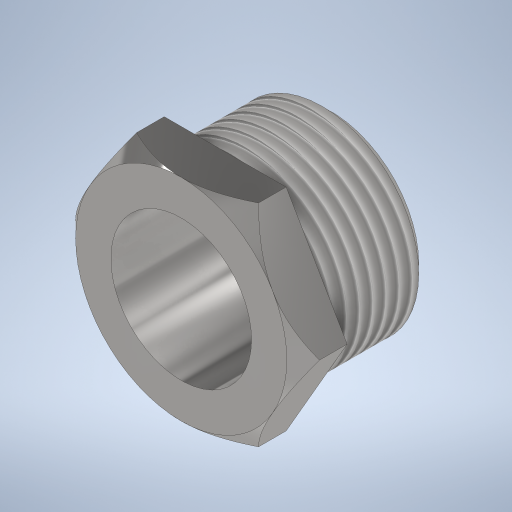
# Autodesk Inventor part: Hex.nut
Saved by Autodesk Inventor 2024 (Build 280153000, 153)
## iProperties
Created: 2024-03-04
Part Number: Hex.nut
Material: Generic
Document SubType Name: Sheet Metal
Designer: MSI-C
Density: 1 g/cm^3
Sheet Metal Rule: Default_mm
Appearance: Steel - Polished
Mass: 3.57819 g
Surface Area: 26.1963 cm^2
Volume: 3.57819 cm^3
Author: MSI-C
Autodesk Inventor part; units mm, degrees
ref_plane "YZ Plane" through (0, 0, 0) normal (1, 0, 0) x (0, 1, 0)
ref_plane "XZ Plane" through (0, 0, 0) normal (0, 1, 0) x (-1, 0, 0)
ref_plane "XY Plane" through (0, 0, 0) normal (0, 0, 1) x (1, 0, 0)
sketch "Sketch1" plane through (0, 0, 0) normal (0, 0, 1) x (1, 0, 0)
  line L0 (-6.9282, -12) -> (-13.8564, 0)
  line L1 (-13.8564, 0) -> (-6.9282, 12)
  line L2 (-6.9282, 12) -> (6.9282, 12)
  line L3 (6.9282, 12) -> (13.8564, 0)
  line L4 (13.8564, 0) -> (6.9282, -12)
  line L5 (6.9282, -12) -> (-6.9282, -12)
  circle A0 centre (0, 0) radius 12
  circle A1 centre (0, 0) radius 7
  dimension "d0" = 24
  dimension "d1" = 24
  dimension "d2" = 14
  constraints: 12 end point, 3 coincident, 2 centre point, 1 horizontal, 13 other
  measures "d0" distance between parallel lines of L5 L2
  measures "d1" diameter of A0
  measures "d2" diameter of A1
extrude "Extrusion1" add sketch "Sketch1" along normal blind 5 contours L0 A0 L5 | L0 L1 A0 | A0 | A0 L4 L5 | L1 L2 A0 | A0 L3 L4 | L2 L3 A0 | A1
sketch "Sketch2" plane through (0, 0, 5) normal (0, 0, 1) x (1, 0, 0)
  circle A0 centre (0, 0) radius 12
  dimension "d5" = 24
  constraints: 1 centre point, 1 coincident
  measures "d5" diameter of A0
extrude "Extrusion2" cut sketch "Sketch2" against normal blind 5 draft 45 keep common part
sketch "Sketch3" plane through (0, 0, 0) normal (0, 0, -1) x (-1, 0, 0)
  circle A0 centre (0, 0) radius 11
  circle A1 centre (0, 0) radius 8
  dimension "d8" = 22
  dimension "d9" = 16
  constraints: 2 centre point, 2 coincident
  measures "d8" diameter of A0
  measures "d9" diameter of A1
extrude "Extrusion3" add sketch "Sketch3" along normal blind 12
extrude "Extrusion4" cut sketch "Sketch3" against normal through all contours A1
thread "Thread1" size "M22x1.5" class "6g" standard "ISO Metric profile" full length
chamfer "Chamfer1" distance 1 angle 45 1 edges at (11, 0, -12)
equation "\"BendRadius\" = Thickness"
equation "\"BendReliefWidth\" = Thickness"
equation "\"BendReliefDepth\" = 0.5 * Thickness"
equation "\"CornerReliefSize\" = 4 * Thickness"
equation "\"MinimumRemnant\" = 2 * Thickness"
equation "\"TransitionRadius\" = BendRadius"
equation "\"JacobiRadiusSize\" = BendRadius"
equation "\"GapSize\" = Thickness"
equation "\"Thickness\" = 0.5"
body "Solid1"
